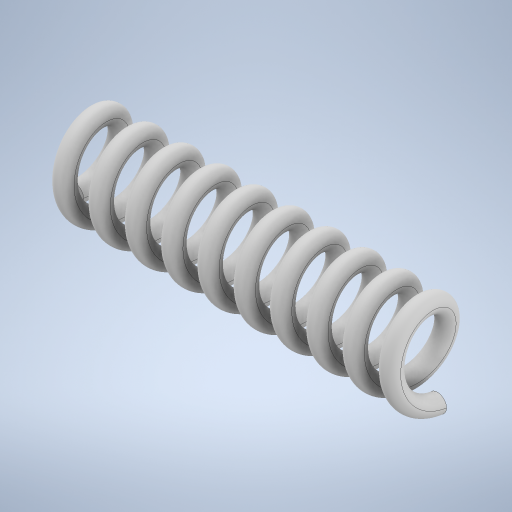
# Autodesk Inventor part: coil_example
Saved by Autodesk Inventor 2024 (Build 280153000, 153)
## iProperties
Created: 2025-02-25
Part Number: coil_example
Material: Generic
Document SubType Name: Modeling
Designer: med287
Density: 1 g/cm^3
Appearance: Default
Author: med287
Autodesk Inventor part; units mm, degrees
ref_plane "YZ Plane" through (0, 0, 0) normal (1, 0, 0) x (0, 1, 0)
ref_plane "XZ Plane" through (0, 0, 0) normal (0, 1, 0) x (-1, 0, 0)
ref_plane "XY Plane" through (0, 0, 0) normal (0, 0, 1) x (1, 0, 0)
sketch "Sketch1" plane through (0, 0, 0) normal (0, 0, 1) x (1, 0, 0)
  circle A0 centre (94.4595, -25.4) radius 6.35
  line L0 (94.4595, 0) -> (-159.5405, 0)
  point P0 (0, 0)
  dimension "d0" = 12.7
  dimension "d1" = 254
  dimension "d2" = 25.4
  constraints: 2 end point, 1 centre point, 1 horizontal
  measures "d0" diameter of A0
  measures "d1" distance of L0.start L0.end
  measures "d2" distance of L0.start A0.centre
coil "Coil1" sketch "Sketch1" operation add axis through (94.4595, 0, 0) along (-1, 0, 0) pitch 25.4 turns 10 hand right
body "Solid1"
